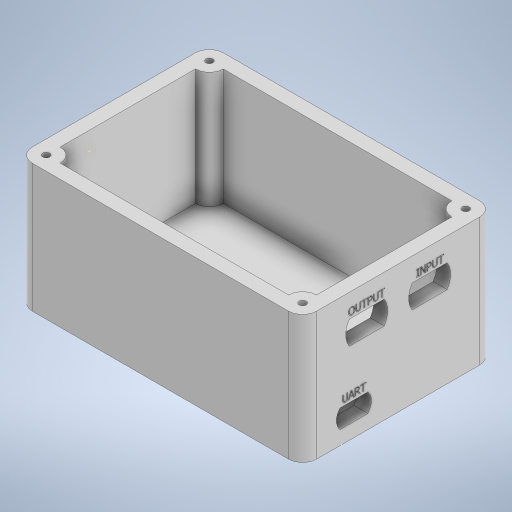
# Autodesk Inventor part: BOX Lurcotte
Saved by Autodesk Inventor 2024 (Build 280153000, 153)
## iProperties
Created: 2025-05-12
Part Number: BOX Lurcotte
Material: Generic
Document SubType Name: Modeling
Designer: chaaa
Density: 1 g/cm^3
Appearance: Default
Author: chaaa
Autodesk Inventor part; units mm, degrees
ref_plane "YZ Plane" through (0, 0, 0) normal (1, 0, 0) x (0, 1, 0)
ref_plane "XZ Plane" through (0, 0, 0) normal (0, 1, 0) x (-1, 0, 0)
ref_plane "XY Plane" through (0, 0, 0) normal (0, 0, 1) x (1, 0, 0)
sketch "Sketch1" plane through (0, 0, 0) normal (0, 1, 0) x (-1, 0, 0)
  point P0 (0, 0)
sketch "Sketch2" plane through (0, 0, 0) normal (0, 1, 0) x (-1, 0, 0)
  line L0 (1.8735, 10.5793) -> (-96.1265, 10.5793)
  line L1 (-102.1265, 4.5793) -> (-102.1265, -53.4207)
  line L2 (-96.1265, -59.4207) -> (1.8735, -59.4207)
  line L3 (7.8735, -53.4207) -> (7.8735, 4.5793)
  line L4 (7.8735, 16.5793) -> (-102.1265, 16.5793)
  line L5 (-108.1265, 10.5793) -> (-108.1265, -59.4207)
  line L6 (-102.1265, -65.4207) -> (7.8735, -65.4207)
  line L7 (13.8735, -59.4207) -> (13.8735, 10.5793)
  circle A0 centre (7.8735, 10.5793) radius 6
  circle A1 centre (7.8735, -59.4207) radius 6
  circle A2 centre (-102.1265, -59.4207) radius 6
  circle A3 centre (-102.1265, 10.5793) radius 6
  circle A4 centre (7.8735, 10.5793) radius 1.5
  circle A5 centre (7.8735, -59.4207) radius 1.5
  circle A6 centre (-102.1265, -59.4207) radius 1.5
  circle A7 centre (-102.1265, 10.5793) radius 1.5
  point P0 (0, 0)
  constraints: 16 end point, 16 point on circle, 8 centre point, 4 coincident, 4 parallel, 3 tangent, 2 perpendicular, 1 horizontal
extrude "Extrusion1" add sketch "Sketch2" along normal blind 5
sketch "Sketch3" plane through (0, 5, 0) normal (0, 1, 0) x (1, 0, 0)
  arc A0 (-7.8735, 65.4207) -> (-13.8735, 59.4207) centre (-7.8735, 59.4207) ccw projected
  line L0 (-7.8735, -16.5793) -> (102.1265, -16.5793) projected
  line L1 (-7.8735, 65.4207) -> (102.1265, 65.4207)
  line L2 (102.1265, -16.5793) -> (-7.8735, -16.5793)
  line L3 (-7.8735, -4.5793) -> (-7.8735, 53.4207)
  line L4 (-13.8735, 59.4207) -> (-13.8735, -10.5793) projected
  line L5 (108.1265, -10.5793) -> (108.1265, 59.4207) projected
  line L6 (-1.8735, -10.5793) -> (96.1265, -10.5793)
  line L7 (108.1265, -10.5793) -> (108.1265, 59.4207)
  line L8 (-13.8735, 59.4207) -> (-13.8735, -10.5793)
  circle A1 centre (-7.8735, 59.4207) radius 6
  circle A2 centre (102.1265, 59.4207) radius 1.5 projected
  circle A3 centre (102.1265, 59.4207) radius 6
  circle A4 centre (102.1265, -10.5793) radius 1.5 projected
  circle A5 centre (102.1265, -10.5793) radius 6
  circle A6 centre (-7.8735, -10.5793) radius 1.5 projected
  circle A7 centre (-7.8735, -10.5793) radius 6
  line L9 (102.1265, 53.4207) -> (102.1265, -4.5793)
  line L10 (96.1265, 59.4207) -> (-1.8735, 59.4207)
  circle A8 centre (-7.8735, 59.4207) radius 1.5 projected
  circle A9 centre (-7.8735, 59.4207) radius 1.5
  point P0 (0, 0)
  constraints: 16 end point, 10 point on circle, 5 centre point, 5 coincident, 4 parallel, 2 horizontal, 2 perpendicular, 1 tangent
extrude "Extrusion2" add sketch "Sketch3" along normal blind 50 contours A1 A0 | L1 A3 L10 A1 | A1 L3 A7 L4 | A3 | A7 | L5 A5 L9 A3 | A7 L6 A5 L0 | A5
sketch "Sketch4" plane through (0, 5, 0) normal (0, 1, 0) x (1, 0, 0)
  arc A0 (102.1265, -4.5793) -> (96.1265, -10.5793) centre (102.1265, -10.5793) ccw projected
  line L0 (96.1265, -10.5793) -> (-1.8735, -10.5793) projected
  point P0 (0, 0)
sketch "Sketch5" plane through (108.1265, 0, 10.5793) normal (1, 0, 0) x (0, 0, -1)
  line L0 (10, 14) -> (22, 14)
  line L1 (22, 6) -> (10, 6)
  line L2 (6, 5) -> (6, 55) projected
  line L3 (6, 5) -> (64, 5) projected
  line L4 (64, 5) -> (64, 55) projected
  line L5 (0, 0) -> (70, 0) projected
  arc A0 (10, 14) -> (10, 6) centre (14.4721, 10) ccw
  arc A1 (22, 6) -> (22, 14) centre (17.5279, 10) ccw
  point P0 (10.5793, 0)
  point P1 (16, 6)
  point P2 (16, 14)
  point P3 (23.5279, 10)
  point P4 (8.4721, 10)
  constraints: 6 point on circle, 4 end point, 2 centre point, 2 midpoint, 1 horizontal, 1 parallel, 1 vertical alignment
extrude "Extrusion3" cut sketch "Sketch5" against normal blind 50
sketch "Sketch7" plane through (0, 55, 0) normal (0, 1, 0) x (1, 0, 0)
  point P0 (0, 0)
sketch "Sketch8" plane through (108.1265, 0, 10.5793) normal (1, 0, 0) x (0, 0, -1)
  line L0 (10.901, 18.1054) -> (21.2158, 18.1054) construction
  line L1 (21.2158, 18.1054) -> (21.2158, 14.9932) construction
  line L2 (21.2158, 14.9932) -> (10.901, 14.9932) construction
  line L3 (10.901, 14.9932) -> (10.901, 18.1054) construction
  spline S0 degree 2 poles (12.2743, 14.9932) (12.0051, 14.9932) (11.6049, 15.134) (11.4641, 15.2748) knots 0 0 0 1 2 2 2
  spline S1 degree 2 poles (11.4641, 15.2748) (11.3036, 15.4329) (11.1727, 15.8775) (11.1727, 16.2035) knots 0 0 0 1 2 2 2
  line L4 (11.1727, 16.2035) -> (11.1727, 18.1054)
  line L5 (11.1727, 18.1054) -> (11.5778, 18.1054)
  line L6 (11.5778, 18.1054) -> (11.5778, 16.2035)
  spline S2 degree 2 poles (11.5778, 16.2035) (11.5778, 15.9911) (11.6321, 15.7046) (11.7087, 15.5885) knots 0 0 0 1 2 2 2
  spline S3 degree 2 poles (11.7087, 15.5885) (11.7902, 15.465) (12.0718, 15.339) (12.2743, 15.339) knots 0 0 0 1 2 2 2
  spline S4 degree 2 poles (12.2743, 15.339) (12.4645, 15.339) (12.7609, 15.465) (12.8424, 15.5885) knots 0 0 0 1 2 2 2
  spline S5 degree 2 poles (12.8424, 15.5885) (12.919, 15.7046) (12.9733, 15.9886) (12.9733, 16.1936) knots 0 0 0 1 2 2 2
  line L7 (12.9733, 16.1936) -> (12.9733, 18.1054)
  line L8 (12.9733, 18.1054) -> (13.3784, 18.1054)
  line L9 (13.3784, 18.1054) -> (13.3784, 16.2035)
  spline S6 degree 2 poles (13.3784, 16.2035) (13.3784, 15.8849) (13.25, 15.4304) (13.0869, 15.2748) knots 0 0 0 1 2 2 2
  spline S7 degree 2 poles (13.0869, 15.2748) (12.9412, 15.1315) (12.5559, 14.9932) (12.2743, 14.9932) knots 0 0 0 1 2 2 2
  line L10 (13.6304, 15.0574) -> (14.6579, 18.1054)
  line L11 (14.6579, 18.1054) -> (15.1568, 18.1054)
  line L12 (15.1568, 18.1054) -> (16.1843, 15.0574)
  line L13 (16.1843, 15.0574) -> (15.757, 15.0574)
  line L14 (15.757, 15.0574) -> (15.4804, 15.9096)
  line L15 (15.4804, 15.9096) -> (14.317, 15.9096)
  line L16 (14.317, 15.9096) -> (14.0404, 15.0574)
  line L17 (14.0404, 15.0574) -> (13.6304, 15.0574)
  line L18 (15.3692, 16.2554) -> (14.8975, 17.6905)
  line L19 (14.8975, 17.6905) -> (14.4282, 16.2554)
  line L20 (14.4282, 16.2554) -> (15.3692, 16.2554)
  line L21 (18.8322, 15.0574) -> (18.3061, 15.0574)
  line L22 (18.3061, 15.0574) -> (17.3428, 16.2702)
  line L23 (17.3428, 16.2702) -> (16.8784, 16.2702)
  line L24 (16.8784, 16.2702) -> (16.8784, 15.0574)
  line L25 (16.8784, 15.0574) -> (16.4733, 15.0574)
  line L26 (16.4733, 15.0574) -> (16.4733, 18.1054)
  line L27 (16.4733, 18.1054) -> (17.2588, 18.1054)
  spline S8 degree 2 poles (17.2588, 18.1054) (17.5206, 18.1054) (17.8738, 18.0486) (18.0344, 17.9449) knots 0 0 0 1 2 2 2
  spline S9 degree 2 poles (18.0344, 17.9449) (18.1949, 17.8411) (18.3802, 17.5176) (18.3802, 17.278) knots 0 0 0 1 2 2 2
  spline S10 degree 2 poles (18.3802, 17.278) (18.3802, 16.9445) (18.0393, 16.4925) (17.7479, 16.3838) knots 0 0 0 1 2 2 2
  line L28 (17.7479, 16.3838) -> (18.8322, 15.0574)
  spline S11 degree 2 poles (17.9578, 17.2459) (17.9578, 17.3793) (17.864, 17.5843) (17.7652, 17.651) knots 0 0 0 1 2 2 2
  spline S12 degree 2 poles (17.7652, 17.651) (17.6787, 17.7078) (17.449, 17.7547) (17.281, 17.7547) knots 0 0 0 1 2 2 2
  line L29 (17.281, 17.7547) -> (16.8784, 17.7547)
  line L30 (16.8784, 17.7547) -> (16.8784, 16.6086)
  line L31 (16.8784, 16.6086) -> (17.2341, 16.6086)
  spline S13 degree 2 poles (17.2341, 16.6086) (17.4095, 16.6086) (17.6886, 16.6704) (17.7849, 16.7667) knots 0 0 0 1 2 2 2
  spline S14 degree 2 poles (17.7849, 16.7667) (17.8738, 16.8507) (17.9578, 17.0878) (17.9578, 17.2459) knots 0 0 0 1 2 2 2
  line L32 (19.7856, 15.0574) -> (19.7856, 17.7448)
  line L33 (19.7856, 17.7448) -> (18.763, 17.7448)
  line L34 (18.763, 17.7448) -> (18.763, 18.1054)
  line L35 (18.763, 18.1054) -> (21.2133, 18.1054)
  line L36 (21.2133, 18.1054) -> (21.2133, 17.7448)
  line L37 (21.2133, 17.7448) -> (20.1907, 17.7448)
  line L38 (20.1907, 17.7448) -> (20.1907, 15.0574)
  line L39 (20.1907, 15.0574) -> (19.7856, 15.0574)
  point P0 (10.5793, 0)
  constraints: 2 other
extrude "Extrusion5" cut sketch "Sketch8" against normal blind 2
sketch "Sketch9" plane through (108.1265, 0, 10.5793) normal (1, 0, 0) x (0, 0, -1)
  point P0 (10.5793, 0)
sketch "Sketch10" plane through (108.1265, 0, 10.5793) normal (1, 0, 0) x (0, 0, -1)
  point P0 (10.5793, 0)
sketch "Sketch11" plane through (108.1265, 0, 10.5793) normal (1, 0, 0) x (0, 0, -1)
  line L0 (14, 45) -> (29, 45)
  line L1 (29, 35) -> (14, 35)
  arc A0 (29, 35) -> (29, 45) centre (21.5, 40) ccw
  arc A1 (14, 45) -> (14, 35) centre (21.5, 40) ccw
  line L2 (6, 5) -> (6, 55) projected
  line L3 (41, 45) -> (56, 45)
  line L4 (56, 35) -> (41, 35)
  arc A2 (56, 35) -> (56, 45) centre (48.5, 40) ccw
  arc A3 (41, 45) -> (41, 35) centre (48.5, 40) ccw
  line L5 (64, 5) -> (64, 55) projected
  line L6 (6, 5) -> (64, 5) projected
  point P0 (10.5793, 0)
  point P1 (56, 40)
  point P2 (48.5, 35)
  point P3 (21.5, 35)
  constraints: 8 end point, 8 point on circle, 4 centre point, 2 horizontal, 2 midpoint, 2 parallel
extrude "Extrusion6" cut sketch "Sketch11" against normal blind 50
sketch "Sketch12" plane through (108.1265, 0, 10.5793) normal (1, 0, 0) x (0, 0, -1)
  line L0 (13.5828, 49.1655) -> (29.2575, 49.1655) construction
  line L1 (29.2575, 49.1655) -> (29.2575, 44.8146) construction
  line L2 (29.2575, 44.8146) -> (13.5828, 44.8146) construction
  line L3 (13.5828, 44.8146) -> (13.5828, 49.1655) construction
  line L4 (42.6906, 49.027) -> (54.564, 49.027) construction
  line L5 (54.564, 49.027) -> (54.564, 45.9148) construction
  line L6 (54.564, 45.9148) -> (42.6906, 45.9148) construction
  line L7 (42.6906, 45.9148) -> (42.6906, 49.027) construction
  line L8 (41, 45) -> (56, 45) projected
  spline S0 degree 2 poles (16.0479, 48.753) (16.2208, 48.5505) (16.4134, 47.9577) (16.4134, 47.5773) knots 0 0 0 1 2 2 2
  spline S1 degree 2 poles (16.4134, 47.5773) (16.4134, 47.2068) (16.2257, 46.6066) (16.0479, 46.404) knots 0 0 0 1 2 2 2
  spline S2 degree 2 poles (16.0479, 46.404) (15.8601, 46.1916) (15.3637, 45.9891) (15.0648, 45.9891) knots 0 0 0 1 2 2 2
  spline S3 degree 2 poles (15.0648, 45.9891) (14.756, 45.9891) (14.262, 46.199) (14.0817, 46.404) knots 0 0 0 1 2 2 2
  spline S4 degree 2 poles (14.0817, 46.404) (13.9064, 46.6066) (13.7186, 47.2018) (13.7186, 47.5773) knots 0 0 0 1 2 2 2
  spline S5 degree 2 poles (13.7186, 47.5773) (13.7186, 47.9601) (13.9088, 48.5431) (14.0842, 48.753) knots 0 0 0 1 2 2 2
  spline S6 degree 2 poles (14.0842, 48.753) (14.262, 48.9556) (14.7585, 49.1655) (15.0648, 49.1655) knots 0 0 0 1 2 2 2
  spline S7 degree 2 poles (15.0648, 49.1655) (15.376, 49.1655) (15.875, 48.9481) (16.0479, 48.753) knots 0 0 0 1 2 2 2
  spline S8 degree 2 poles (15.9911, 47.5773) (15.9911, 47.8786) (15.8601, 48.3455) (15.7416, 48.4986) knots 0 0 0 1 2 2 2
  spline S9 degree 2 poles (15.7416, 48.4986) (15.6206, 48.6567) (15.2797, 48.8148) (15.0673, 48.8148) knots 0 0 0 1 2 2 2
  spline S10 degree 2 poles (15.0673, 48.8148) (14.8474, 48.8148) (14.5165, 48.6616) (14.3905, 48.4986) knots 0 0 0 1 2 2 2
  spline S11 degree 2 poles (14.3905, 48.4986) (14.2695, 48.343) (14.141, 47.8737) (14.141, 47.5773) knots 0 0 0 1 2 2 2
  spline S12 degree 2 poles (14.141, 47.5773) (14.141, 46.9771) (14.6449, 46.3398) (15.0673, 46.3398) knots 0 0 0 1 2 2 2
  spline S13 degree 2 poles (15.0673, 46.3398) (15.4896, 46.3398) (15.9911, 46.9771) (15.9911, 47.5773) knots 0 0 0 1 2 2 2
  spline S14 degree 2 poles (17.9226, 45.9891) (17.6534, 45.9891) (17.2532, 46.1299) (17.1124, 46.2707) knots 0 0 0 1 2 2 2
  spline S15 degree 2 poles (17.1124, 46.2707) (16.9519, 46.4287) (16.821, 46.8733) (16.821, 47.1994) knots 0 0 0 1 2 2 2
  line L9 (16.821, 47.1994) -> (16.821, 49.1013)
  line L10 (16.821, 49.1013) -> (17.2261, 49.1013)
  line L11 (17.2261, 49.1013) -> (17.2261, 47.1994)
  spline S16 degree 2 poles (17.2261, 47.1994) (17.2261, 46.987) (17.2804, 46.7004) (17.357, 46.5843) knots 0 0 0 1 2 2 2
  spline S17 degree 2 poles (17.357, 46.5843) (17.4385, 46.4608) (17.7201, 46.3349) (17.9226, 46.3349) knots 0 0 0 1 2 2 2
  spline S18 degree 2 poles (17.9226, 46.3349) (18.1128, 46.3349) (18.4092, 46.4608) (18.4907, 46.5843) knots 0 0 0 1 2 2 2
  spline S19 degree 2 poles (18.4907, 46.5843) (18.5673, 46.7004) (18.6216, 46.9845) (18.6216, 47.1895) knots 0 0 0 1 2 2 2
  line L12 (18.6216, 47.1895) -> (18.6216, 49.1013)
  line L13 (18.6216, 49.1013) -> (19.0267, 49.1013)
  line L14 (19.0267, 49.1013) -> (19.0267, 47.1994)
  spline S20 degree 2 poles (19.0267, 47.1994) (19.0267, 46.8807) (18.8983, 46.4263) (18.7352, 46.2707) knots 0 0 0 1 2 2 2
  spline S21 degree 2 poles (18.7352, 46.2707) (18.5895, 46.1274) (18.2042, 45.9891) (17.9226, 45.9891) knots 0 0 0 1 2 2 2
  line L15 (20.3185, 46.0533) -> (20.3185, 48.7407)
  line L16 (20.3185, 48.7407) -> (19.2959, 48.7407)
  line L17 (19.2959, 48.7407) -> (19.2959, 49.1013)
  line L18 (19.2959, 49.1013) -> (21.7462, 49.1013)
  line L19 (21.7462, 49.1013) -> (21.7462, 48.7407)
  line L20 (21.7462, 48.7407) -> (20.7236, 48.7407)
  line L21 (20.7236, 48.7407) -> (20.7236, 46.0533)
  line L22 (20.7236, 46.0533) -> (20.3185, 46.0533)
  spline S22 degree 2 poles (23.9816, 48.1824) (23.9816, 47.9848) (23.8408, 47.6292) (23.7148, 47.5057) knots 0 0 0 1 2 2 2
  spline S23 degree 2 poles (23.7148, 47.5057) (23.5567, 47.35) (23.1294, 47.1895) (22.8034, 47.1895) knots 0 0 0 1 2 2 2
  line L23 (22.8034, 47.1895) -> (22.46, 47.1895)
  line L24 (22.46, 47.1895) -> (22.46, 46.0533)
  line L25 (22.46, 46.0533) -> (22.0549, 46.0533)
  line L26 (22.0549, 46.0533) -> (22.0549, 49.1013)
  line L27 (22.0549, 49.1013) -> (22.8206, 49.1013)
  spline S24 degree 2 poles (22.8206, 49.1013) (23.0924, 49.1013) (23.4727, 49.0124) (23.6185, 48.9111) knots 0 0 0 1 2 2 2
  spline S25 degree 2 poles (23.6185, 48.9111) (23.7889, 48.795) (23.9816, 48.4369) (23.9816, 48.1824) knots 0 0 0 1 2 2 2
  spline S26 degree 2 poles (23.5592, 48.1701) (23.5592, 48.3282) (23.4505, 48.5604) (23.3394, 48.6345) knots 0 0 0 1 2 2 2
  spline S27 degree 2 poles (23.3394, 48.6345) (23.243, 48.6987) (22.9861, 48.7505) (22.7959, 48.7505) knots 0 0 0 1 2 2 2
  line L28 (22.7959, 48.7505) -> (22.46, 48.7505)
  line L29 (22.46, 48.7505) -> (22.46, 47.5353)
  line L30 (22.46, 47.5353) -> (22.7367, 47.5353)
  spline S28 degree 2 poles (22.7367, 47.5353) (22.9837, 47.5353) (23.2875, 47.6143) (23.3863, 47.7181) knots 0 0 0 1 2 2 2
  spline S29 degree 2 poles (23.3863, 47.7181) (23.4777, 47.8095) (23.5592, 48.0244) (23.5592, 48.1701) knots 0 0 0 1 2 2 2
  spline S30 degree 2 poles (25.4315, 45.9891) (25.1622, 45.9891) (24.7621, 46.1299) (24.6213, 46.2707) knots 0 0 0 1 2 2 2
  spline S31 degree 2 poles (24.6213, 46.2707) (24.4607, 46.4287) (24.3298, 46.8733) (24.3298, 47.1994) knots 0 0 0 1 2 2 2
  line L31 (24.3298, 47.1994) -> (24.3298, 49.1013)
  line L32 (24.3298, 49.1013) -> (24.7349, 49.1013)
  line L33 (24.7349, 49.1013) -> (24.7349, 47.1994)
  spline S32 degree 2 poles (24.7349, 47.1994) (24.7349, 46.987) (24.7893, 46.7004) (24.8658, 46.5843) knots 0 0 0 1 2 2 2
  spline S33 degree 2 poles (24.8658, 46.5843) (24.9473, 46.4608) (25.2289, 46.3349) (25.4315, 46.3349) knots 0 0 0 1 2 2 2
  spline S34 degree 2 poles (25.4315, 46.3349) (25.6216, 46.3349) (25.918, 46.4608) (25.9996, 46.5843) knots 0 0 0 1 2 2 2
  spline S35 degree 2 poles (25.9996, 46.5843) (26.0761, 46.7004) (26.1305, 46.9845) (26.1305, 47.1895) knots 0 0 0 1 2 2 2
  line L34 (26.1305, 47.1895) -> (26.1305, 49.1013)
  line L35 (26.1305, 49.1013) -> (26.5356, 49.1013)
  line L36 (26.5356, 49.1013) -> (26.5356, 47.1994)
  spline S36 degree 2 poles (26.5356, 47.1994) (26.5356, 46.8807) (26.4071, 46.4263) (26.2441, 46.2707) knots 0 0 0 1 2 2 2
  spline S37 degree 2 poles (26.2441, 46.2707) (26.0984, 46.1274) (25.713, 45.9891) (25.4315, 45.9891) knots 0 0 0 1 2 2 2
  line L37 (27.8274, 46.0533) -> (27.8274, 48.7407)
  line L38 (27.8274, 48.7407) -> (26.8048, 48.7407)
  line L39 (26.8048, 48.7407) -> (26.8048, 49.1013)
  line L40 (26.8048, 49.1013) -> (29.255, 49.1013)
  line L41 (29.255, 49.1013) -> (29.255, 48.7407)
  line L42 (29.255, 48.7407) -> (28.2325, 48.7407)
  line L43 (28.2325, 48.7407) -> (28.2325, 46.0533)
  line L44 (28.2325, 46.0533) -> (27.8274, 46.0533)
  line L45 (44.0615, 45.979) -> (42.8808, 45.979)
  line L46 (42.8808, 45.979) -> (42.8808, 46.2903)
  line L47 (42.8808, 46.2903) -> (43.2686, 46.2903)
  line L48 (43.2686, 46.2903) -> (43.2686, 48.7158)
  line L49 (43.2686, 48.7158) -> (42.8808, 48.7158)
  line L50 (42.8808, 48.7158) -> (42.8808, 49.027)
  line L51 (42.8808, 49.027) -> (44.0615, 49.027)
  line L52 (44.0615, 49.027) -> (44.0615, 48.7158)
  line L53 (44.0615, 48.7158) -> (43.6737, 48.7158)
  line L54 (43.6737, 48.7158) -> (43.6737, 46.2903)
  line L55 (43.6737, 46.2903) -> (44.0615, 46.2903)
  line L56 (44.0615, 46.2903) -> (44.0615, 45.979)
  line L57 (46.7439, 45.979) -> (46.2895, 45.979)
  line L58 (46.2895, 45.979) -> (44.9408, 48.6071)
  line L59 (44.9408, 48.6071) -> (44.9408, 45.979)
  line L60 (44.9408, 45.979) -> (44.5629, 45.979)
  line L61 (44.5629, 45.979) -> (44.5629, 49.027)
  line L62 (44.5629, 49.027) -> (45.1384, 49.027)
  line L63 (45.1384, 49.027) -> (46.366, 46.6138)
  line L64 (46.366, 46.6138) -> (46.366, 49.027)
  line L65 (46.366, 49.027) -> (46.7439, 49.027)
  line L66 (46.7439, 49.027) -> (46.7439, 45.979)
  spline S38 degree 2 poles (49.2881, 48.1082) (49.2881, 47.9106) (49.1473, 47.5549) (49.0213, 47.4314) knots 0 0 0 1 2 2 2
  spline S39 degree 2 poles (49.0213, 47.4314) (48.8632, 47.2758) (48.4359, 47.1152) (48.1099, 47.1152) knots 0 0 0 1 2 2 2
  line L67 (48.1099, 47.1152) -> (47.7665, 47.1152)
  line L68 (47.7665, 47.1152) -> (47.7665, 45.979)
  line L69 (47.7665, 45.979) -> (47.3614, 45.979)
  line L70 (47.3614, 45.979) -> (47.3614, 49.027)
  line L71 (47.3614, 49.027) -> (48.1271, 49.027)
  spline S40 degree 2 poles (48.1271, 49.027) (48.3988, 49.027) (48.7792, 48.9381) (48.925, 48.8368) knots 0 0 0 1 2 2 2
  spline S41 degree 2 poles (48.925, 48.8368) (49.0954, 48.7207) (49.2881, 48.3626) (49.2881, 48.1082) knots 0 0 0 1 2 2 2
  spline S42 degree 2 poles (48.8657, 48.0958) (48.8657, 48.2539) (48.757, 48.4861) (48.6458, 48.5602) knots 0 0 0 1 2 2 2
  spline S43 degree 2 poles (48.6458, 48.5602) (48.5495, 48.6244) (48.2926, 48.6763) (48.1024, 48.6763) knots 0 0 0 1 2 2 2
  line L72 (48.1024, 48.6763) -> (47.7665, 48.6763)
  line L73 (47.7665, 48.6763) -> (47.7665, 47.461)
  line L74 (47.7665, 47.461) -> (48.0432, 47.461)
  spline S44 degree 2 poles (48.0432, 47.461) (48.2902, 47.461) (48.594, 47.5401) (48.6928, 47.6438) knots 0 0 0 1 2 2 2
  spline S45 degree 2 poles (48.6928, 47.6438) (48.7842, 47.7352) (48.8657, 47.9501) (48.8657, 48.0958) knots 0 0 0 1 2 2 2
  spline S46 degree 2 poles (50.738, 45.9148) (50.4687, 45.9148) (50.0686, 46.0556) (49.9278, 46.1964) knots 0 0 0 1 2 2 2
  spline S47 degree 2 poles (49.9278, 46.1964) (49.7672, 46.3545) (49.6363, 46.7991) (49.6363, 47.1251) knots 0 0 0 1 2 2 2
  line L75 (49.6363, 47.1251) -> (49.6363, 49.027)
  line L76 (49.6363, 49.027) -> (50.0414, 49.027)
  line L77 (50.0414, 49.027) -> (50.0414, 47.1251)
  spline S48 degree 2 poles (50.0414, 47.1251) (50.0414, 46.9127) (50.0957, 46.6262) (50.1723, 46.5101) knots 0 0 0 1 2 2 2
  spline S49 degree 2 poles (50.1723, 46.5101) (50.2538, 46.3866) (50.5354, 46.2606) (50.738, 46.2606) knots 0 0 0 1 2 2 2
  spline S50 degree 2 poles (50.738, 46.2606) (50.9281, 46.2606) (51.2245, 46.3866) (51.3061, 46.5101) knots 0 0 0 1 2 2 2
  spline S51 degree 2 poles (51.3061, 46.5101) (51.3826, 46.6262) (51.437, 46.9102) (51.437, 47.1152) knots 0 0 0 1 2 2 2
  line L78 (51.437, 47.1152) -> (51.437, 49.027)
  line L79 (51.437, 49.027) -> (51.842, 49.027)
  line L80 (51.842, 49.027) -> (51.842, 47.1251)
  spline S52 degree 2 poles (51.842, 47.1251) (51.842, 46.8065) (51.7136, 46.352) (51.5506, 46.1964) knots 0 0 0 1 2 2 2
  spline S53 degree 2 poles (51.5506, 46.1964) (51.4049, 46.0531) (51.0195, 45.9148) (50.738, 45.9148) knots 0 0 0 1 2 2 2
  line L81 (53.1339, 45.979) -> (53.1339, 48.6664)
  line L82 (53.1339, 48.6664) -> (52.1113, 48.6664)
  line L83 (52.1113, 48.6664) -> (52.1113, 49.027)
  line L84 (52.1113, 49.027) -> (54.5615, 49.027)
  line L85 (54.5615, 49.027) -> (54.5615, 48.6664)
  line L86 (54.5615, 48.6664) -> (53.539, 48.6664)
  line L87 (53.539, 48.6664) -> (53.539, 45.979)
  line L88 (53.539, 45.979) -> (53.1339, 45.979)
  point P0 (10.5793, 0)
  point P1 (48.5, 45)
  point P2 (48.6273, 45.9148)
  constraints: 2 midpoint, 4 other
extrude "Extrusion7" cut sketch "Sketch12" against normal blind 2
body "Solid1"
